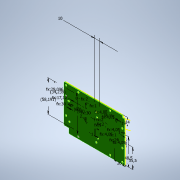
# Autodesk Inventor part: NCU_PCB
Saved by Autodesk Inventor 2021 (Build 250183000, 183)
## iProperties
Created: 2020-02-27
Part Number: NCU_PCB
Material: Generic
Document SubType Name: Modeling
Designer: lgnds
Density: 1 g/cm^3
Appearance: Default
Author: lgnds
Autodesk Inventor part; units mm, degrees
ref_plane "YZ Plane" through (0, 0, 0) normal (1, 0, 0) x (0, 1, 0)
ref_plane "XZ Plane" through (0, 0, 0) normal (0, 1, 0) x (-1, 0, 0)
ref_plane "XY Plane" through (0, 0, 0) normal (0, 0, 1) x (1, 0, 0)
sketch "Sketch1" plane through (0, 0, 0) normal (0, 0, 1) x (1, 0, 0)
  line L0 (-56.1965, -39.8485) -> (56.1965, -39.8485)
  line L1 (56.1965, -39.8485) -> (56.1965, 39.8485)
  line L2 (56.1965, 39.8485) -> (-56.1965, 39.8485)
  line L3 (-56.1965, 39.8485) -> (-56.1965, -39.8485)
  line L4 (-56.1965, -39.8485) -> (56.1965, 39.8485) construction
  line L5 (56.1965, -39.8485) -> (-56.1965, 39.8485) construction
  line L6 (-51.6965, -49.6139) -> (-51.6965, 54.5718) construction
  line L7 (0, -76.4005) -> (0, 76.4005) construction
  line L8 (-3185.9994, 0) -> (3185.9994, 0) construction
  line L9 (-51.6965, 49.6139) -> (-51.6965, -54.5718) construction
  circle A0 centre (-51.6965, -12.8485) radius 1.6
  line L10 (51.6965, -49.6139) -> (51.6965, 54.5718) construction
  line L11 (3185.9994, 0) -> (-3185.9994, 0) construction
  line L12 (51.6965, 49.6139) -> (51.6965, -54.5718) construction
  line L13 (-80.9041, 2.7045) -> (105.3578, 2.7045) construction
  line L14 (51.6965, -49.6139) -> (51.6965, 54.5718) construction
  line L15 (51.6965, 49.6139) -> (51.6965, -54.5718) construction
  circle A1 centre (51.6965, -12.8485) radius 1.6
  circle A2 centre (-51.6965, 18.2575) radius 1.6
  circle A3 centre (51.6965, 18.2575) radius 1.6
  line L16 (-83.6423, -35.3485) -> (68.6664, -35.3485) construction
  circle A4 centre (-29.1965, -35.3485) radius 1.6
  circle A5 centre (29.1965, -35.3485) radius 1.6
  circle A6 centre (-29.1965, 35.3485) radius 1.6
  circle A7 centre (29.1965, 35.3485) radius 1.6
  point P0 (0, 0)
  dimension "d0" = 112.393
  dimension "d1" = 79.697
  dimension "d2" = 4.5
  dimension "d13" = 27
  dimension "d14" = 3.2
  dimension "d15" = 31.106
  dimension "d16" = 4.5
  dimension "d17" = 3.2
  dimension "d18" = 3.2
  dimension "d20" = 27
  dimension "d21" = 27
  constraints: 30 end point, 13 symmetric about line, 8 centre point, 4 point on line, 3 horizontal, 2 midpoint, 2 parallel, 1 perpendicular, 1 vertical, 5 other
  measures "d0" distance of L1.end L2.end
  measures "d1" distance of L0.end L1.end
  measures "d2" distance between parallel lines of L3 L6
  measures "d13" distance from line of L0 A0.centre
  measures "d14" diameter of A0
  measures "d15" distance of A0.centre A2.centre
  measures "d16" distance between parallel lines of L0 L16
  measures "d17" diameter of A4
  measures "d18" diameter of A5
  measures "d20" distance from line of L3 A4.centre
  measures "d21" distance from line of L1 A5.centre
extrude "Extrusion3" add sketch "Sketch1" along normal blind 1.6
thicken "Thicken1" operation add thickness 0.75 both sides no extend neighbours yes toward (0, 1, 0) faces at (-18.7322, -39.8485, 1.0667) (56.1965, -13.2828, 0.5333) (18.7322, 39.8485, 0.5333) (-56.1965, 13.2828, 0.5333)
sketch "Sketch6" plane through (0, 0, 0) normal (0, 0, -1) x (-1, 0, 0)
  circle A0 centre (-5.3535, 12.3015) radius 1.6
  circle A1 centre (46.7956, 12.6015) radius 1.6
  circle A2 centre (45.4465, -19.5985) radius 1.6
  circle A3 centre (-6.7035, -19.8985) radius 1.6
  line L0 (55.4465, 39.0985) -> (55.4465, -39.0985) projected
  line L1 (55.4465, -39.0985) -> (-55.4465, -39.0985) projected
  point P0 (0, 0)
  dimension "d94" = 3.2
  dimension "d95" = 3.2
  dimension "d96" = 3.2
  dimension "d97" = 3.2
  dimension "d98" = 52.15
  dimension "d99" = 52.15
  dimension "d100" = 32.2
  dimension "d102" = 0.3
  dimension "d103" = 32.2
  dimension "d106" = 1.35
  dimension "d107" = 10
  dimension "d108" = 19.5
  constraints: 4 centre point
  measures "d94" diameter of A0
  measures "d95" diameter of A1
  measures "d96" diameter of A3
  measures "d97" diameter of A2
  measures "d98" distance of A0.centre A1.centre
  measures "d99" horizontal distance of A2.centre A3.centre
  measures "d100" vertical distance of A0.centre A3.centre
  measures "d102" vertical distance of A0.centre A1.centre
  measures "d103" vertical distance of A2.centre A1.centre
  measures "d106" horizontal distance of A3.centre A0.centre
  measures "d107" distance from line of L0 A2.centre
  measures "d108" distance from line of L1 A2.centre
extrude "Extrusion6" cut sketch "Sketch6" against normal up to next
sketch "Sketch7" plane through (0, 0, 0) normal (0, 0, -1) x (-1, 0, 0)
  line L0 (-42.5, 39.529) -> (-42.5, 7.5447)
  line L1 (-55.1988, 25) -> (-33.1451, 25)
  line L2 (-55.4465, -39.0985) -> (-55.4465, 39.0985) projected
  line L3 (-55.4465, 39.0985) -> (55.4465, 39.0985) projected
  point P0 (0, 0)
  dimension "d111" = 25
  dimension "d112" = 42.5
  constraints: 4 end point, 1 horizontal, 1 vertical
  measures "d111" distance from line of point (0, 0) L1
  measures "d112" distance from line of point (0, 0) L0
fillet "Fillet3" radius 1 2 edges at (55.4465, -39.0985, 0.8) (-55.4465, 39.0985, 0.8)
sketch "Sketch8" plane through (0, 0, 0) normal (0, 0, -1) x (-1, 0, 0)
  line L0 (55.4465, -39.0985) -> (-54.4465, -39.0985) projected
  line L1 (55.4465, -39.0985) -> (46.4465, -39.0985)
  line L2 (46.4465, -39.0985) -> (46.4465, -30.0985)
  line L3 (46.4465, -30.0985) -> (55.4465, -30.0985)
  line L4 (55.4465, -30.0985) -> (55.4465, -39.0985)
  line L5 (-55.4465, 39.0985) -> (-51.6965, 39.0985)
  line L6 (-51.6965, 39.0985) -> (-51.6965, 35.3485)
  line L7 (-51.6965, 35.3485) -> (-55.4465, 35.3485)
  line L8 (-55.4465, 35.3485) -> (-55.4465, 39.0985)
  point P0 (0, 0)
  dimension "d119" = 9
  dimension "d120" = 9
  dimension "d130" = 3.75
  dimension "d131" = 3.75
  constraints: 16 end point, 4 parallel, 2 horizontal, 2 perpendicular
  measures "d119" distance of L2.end L3.end
  measures "d120" distance of L1.end L2.end
  measures "d130" distance of L5.end L6.end
  measures "d131" distance of L6.end L7.end
extrude "Extrusion7" cut sketch "Sketch8" against normal blind 10
fillet "Fillet5" radius 1 6 edges at (-55.4465, -30.0985, 0.8) (-46.4465, -30.0985, 0.8) (-46.4465, -39.0985, 0.8) (51.6965, 39.0985, 0.8) (51.6965, 35.3485, 0.8) (55.4465, 35.3485, 0.8)
sketch "Sketch9" plane through (0, 0, 0) normal (0, 0, -1) x (-1, 0, 0)
  circle A0 centre (-51.6965, -12.8485) radius 1.6 construction
  circle A1 centre (-29.1965, -35.3485) radius 1.6 construction
  line L0 (-51.6965, -12.8485) -> (-51.6965, -35.3485) construction
  line L1 (-51.6965, -35.3485) -> (-29.1965, -35.3485) construction
  circle A2 centre (29.1965, 35.3485) radius 1.6 construction
  circle A3 centre (51.6965, 18.2575) radius 1.6 construction
  line L2 (29.1965, 35.3485) -> (51.6965, 35.3485) construction
  line L3 (51.6965, 35.3485) -> (51.6965, 18.2575) construction
  circle A4 centre (51.6965, 35.3485) radius 1.6
  circle A5 centre (-51.6965, -35.3485) radius 1.6
  point P0 (0, 0)
  dimension "d124" = 3.2
  dimension "d125" = 3.2
  dimension "d126" = 3.2
  constraints: 8 end point, 2 centre point, 2 coincident, 2 perpendicular, 1 horizontal, 1 vertical
  measures "d124" diameter of A0
  measures "d125" diameter of A5
  measures "d126" diameter of A4
extrude "Extrusion8" cut sketch "Sketch9" against normal up to next
sketch "Sketch10" plane through (0, 0, 0) normal (0, 0, -1) x (-1, 0, 0)
  circle A0 centre (-3.8035, -27.8485) radius 1.6
  line L0 (55.4465, 38.0985) -> (55.4465, -29.0985) projected
  circle A1 centre (-29.1965, 35.3485) radius 1.6 projected
  line L1 (45.4465, -39.0985) -> (-54.4465, -39.0985) projected
  line L2 (-3.8035, -27.8485) -> (-3.8035, 21.0509) construction
  circle A2 centre (-3.8035, 20.1515) radius 1.6
  point P0 (0, 0)
  dimension "d132" = 59.25
  dimension "d133" = 3.2
  dimension "d134" = 3.2
  dimension "d135" = 11.25
  dimension "d136" = 3.2
  dimension "d137" = 48
  constraints: 2 centre point, 2 end point, 1 point on line, 1 vertical
  measures "d132" distance from line of L0 L2.start
  measures "d133" diameter of A0
  measures "d134" diameter of A1
  measures "d135" distance from line of L1 L2.start
  measures "d136" diameter of A2
  measures "d137" distance of A2.centre L2.start
extrude "Extrusion9" cut sketch "Sketch10" against normal up to next contours A0 | A2
sketch "CLIPS" plane through (0, 0, 0) normal (0, 0, -1) x (-1, 0, 0)
  line L0 (-55.4465, -38.0985) -> (-55.4465, 34.3485) projected
  line L1 (-55.4465, 9.4015) -> (-38.9219, 9.4015)
  line L2 (-49.4465, 9.4015) -> (-49.4465, 1.3015)
  line L3 (-36.4465, 30.4761) -> (-36.4465, 19.7209)
  line L4 (-36.4465, 25.0985) -> (-31.2482, 25.0985)
  line L5 (-50.6965, 39.0985) -> (54.4465, 39.0985) projected
  line L6 (1, 31.0993) -> (1, 19.0977)
  line L7 (1, 25.0985) -> (9.1, 25.0985)
  line L8 (-39.6026, -3.5985) -> (-31.2904, -3.5985)
  line L9 (-35.4465, -3.5985) -> (-35.4465, -8.8428)
  line L10 (-12.8208, -3.5985) -> (-5.1792, -3.5985)
  line L11 (-9, -3.5985) -> (-9, -9.7701)
  circle A0 centre (-49.4465, 9.4015) radius 0.5
  circle A1 centre (-35.4465, -3.5985) radius 0.5
  circle A2 centre (-9, -3.5985) radius 0.5
  circle A3 centre (1, 25.0985) radius 0.5
  circle A4 centre (-36.4465, 25.0985) radius 0.5
  circle A5 centre (-49.4465, 5.3515) radius 1
  circle A6 centre (-35.4465, -7.6485) radius 1
  circle A7 centre (-9, -7.6485) radius 1
  circle A8 centre (5.05, 25.0985) radius 1
  circle A9 centre (-32.3965, 25.0985) radius 1
  line L12 (-28.3465, 25.9985) -> (-28.3465, 24.1985) projected
  line L13 (45.4465, -39.0985) -> (-54.4465, -39.0985) projected
  point P0 (0, 0)
  dimension "d140" = 6
  dimension "d141" = 19
  dimension "d142" = 14
  dimension "d143" = 1
  dimension "d144" = 0
  dimension "d145" = 10
  dimension "d146" = 0
  dimension "d147" = 1
  dimension "d148" = 1
  dimension "d149" = 1
  dimension "d150" = 1
  dimension "d151" = 1
  dimension "d157" = 2
  dimension "d158" = 2
  dimension "d159" = 2
  dimension "d160" = 2
  dimension "d161" = 2
  dimension "d162" = 8.1
  dimension "d163" = 4.05
  dimension "d164" = 4.05
  dimension "d165" = 4.05
  dimension "d166" = 4.05
  dimension "d167" = 4.05
  dimension "d168" = 35.5
  dimension "d169" = 48.5
  dimension "d170" = 20
  constraints: 20 end point, 10 centre point, 6 midpoint, 5 coincident, 5 horizontal, 5 point on line, 5 vertical
  measures "d140" distance between parallel lines of L0 L2
  measures "d141" distance between parallel lines of L0 L3
  measures "d142" distance between parallel lines of L5 L4
  measures "d143" distance from line of L6 point (0, 0)
  measures "d144" distance between parallel lines of L4 L7
  measures "d145" distance between parallel lines of L11 L6
  measures "d146" distance between parallel lines of L10 L8
  measures "d147" diameter of A0
  measures "d148" diameter of A1
  measures "d149" diameter of A2
  measures "d150" diameter of A3
  measures "d151" diameter of A4
  measures "d157" diameter of A9
  measures "d158" diameter of A8
  measures "d159" diameter of A7
  measures "d160" diameter of A6
  measures "d161" diameter of A5
  measures "d162" distance between parallel lines of L12 L3
  measures "d163" distance from line of L12 A9.centre
  measures "d164" distance from line of L1 A5.centre
  measures "d165" distance from line of L8 A6.centre
  measures "d166" distance from line of L10 A7.centre
  measures "d167" distance from line of L6 A8.centre
  measures "d168" distance between parallel lines of L13 L8
  measures "d169" distance between parallel lines of L13 L1
  measures "d170" distance between parallel lines of L0 L9
sketch "OUTLINE" plane through (0, 0, 0) normal (0, 0, -1) x (-1, 0, 0)
  line L0 (-50.6965, 39.0985) -> (54.4465, 39.0985) projected
  arc A0 (-50.6965, 39.0985) -> (-51.6965, 38.0985) centre (-50.6965, 38.0985) ccw projected
  line L1 (-51.6965, 38.0985) -> (-51.6965, 36.3485) projected
  arc A1 (-52.6965, 35.3485) -> (-51.6965, 36.3485) centre (-52.6965, 36.3485) ccw projected
  line L2 (-52.6965, 35.3485) -> (-54.4465, 35.3485) projected
  arc A2 (-54.4465, 35.3485) -> (-55.4465, 34.3485) centre (-54.4465, 34.3485) ccw projected
  line L3 (-55.4465, -38.0985) -> (-55.4465, 34.3485) projected
  arc A3 (-55.4465, -38.0985) -> (-54.4465, -39.0985) centre (-54.4465, -38.0985) ccw projected
  line L4 (45.4465, -39.0985) -> (-54.4465, -39.0985) projected
  arc A4 (45.4465, -39.0985) -> (46.4465, -38.0985) centre (45.4465, -38.0985) ccw projected
  line L5 (46.4465, -38.0985) -> (46.4465, -31.0985) projected
  arc A5 (47.4465, -30.0985) -> (46.4465, -31.0985) centre (47.4465, -31.0985) ccw projected
  line L6 (47.4465, -30.0985) -> (54.4465, -30.0985) projected
  arc A6 (54.4465, -30.0985) -> (55.4465, -29.0985) centre (54.4465, -29.0985) ccw projected
  line L7 (55.4465, 38.0985) -> (55.4465, -29.0985) projected
  arc A7 (55.4465, 38.0985) -> (54.4465, 39.0985) centre (54.4465, 38.0985) ccw projected
  point P0 (0, 0)
sketch "EXTRA" plane through (0, 0, 0) normal (0, 0, -1) x (-1, 0, 0)
  circle A0 centre (-29.1965, 35.3485) radius 1.6 projected
  circle A1 centre (-51.6965, 18.2575) radius 1.6 projected
  circle A2 centre (-51.6965, -12.8485) radius 1.6 projected
  circle A3 centre (-51.6965, -35.3485) radius 1.6 projected
  circle A4 centre (-29.1965, -35.3485) radius 1.6 projected
  circle A5 centre (-3.8035, -27.8485) radius 1.5 projected
  circle A6 centre (29.1965, -35.3485) radius 1.5 projected
  circle A7 centre (45.4465, -19.5985) radius 1.6 projected
  circle A8 centre (51.6965, -12.8485) radius 1.5 projected
  circle A9 centre (46.7965, 12.6015) radius 1.6 projected
  circle A10 centre (51.6965, 18.2575) radius 1.5 projected
  circle A11 centre (51.6965, 35.3485) radius 1.6 projected
  circle A12 centre (29.1965, 35.3485) radius 1.6 projected
  circle A13 centre (-5.3535, 12.3015) radius 1.6 projected
  circle A14 centre (-6.7035, -19.8985) radius 1.6 projected
  circle A15 centre (46.7965, 12.6015) radius 1.6 projected
  circle A16 centre (-6.7035, -19.8985) radius 1.6 projected
  circle A17 centre (-5.3535, 12.3015) radius 1.6 projected
  circle A18 centre (45.4465, -19.5985) radius 1.6 projected
  arc A19 (0.0465, -30.6485) -> (3.0465, -33.6485) centre (3.0465, -30.6485) ccw projected
  line L0 (3.0465, -33.6485) -> (37.0465, -33.6485) projected
  arc A20 (37.0465, -33.6485) -> (40.0465, -30.6485) centre (37.0465, -30.6485) ccw projected
  line L1 (40.0465, -30.6485) -> (40.0465, -26.6485) projected
  arc A21 (43.0465, -23.6485) -> (40.0465, -26.6485) centre (43.0465, -26.6485) ccw projected
  line L2 (43.0465, -23.6485) -> (47.0465, -23.6485) projected
  arc A22 (47.0465, -23.6485) -> (50.0465, -20.6485) centre (47.0465, -20.6485) ccw projected
  line L3 (50.0465, -20.6485) -> (50.0465, 13.3515) projected
  arc A23 (50.0465, 13.3515) -> (47.0465, 16.3515) centre (47.0465, 13.3515) ccw projected
  line L4 (47.0465, 16.3515) -> (43.0465, 16.3515) projected
  arc A24 (40.0465, 19.3515) -> (43.0465, 16.3515) centre (43.0465, 19.3515) ccw projected
  line L5 (40.0465, 19.3515) -> (40.0465, 23.3515) projected
  arc A25 (40.0465, 23.3515) -> (37.0465, 26.3515) centre (37.0465, 23.3515) ccw projected
  line L6 (37.0465, 26.3515) -> (3.0465, 26.3515) projected
  arc A26 (3.0465, 26.3515) -> (0.0465, 23.3515) centre (3.0465, 23.3515) ccw projected
  line L7 (0.0465, 23.3515) -> (0.0465, 19.3515) projected
  arc A27 (-2.9535, 16.3515) -> (0.0465, 19.3515) centre (-2.9535, 19.3515) ccw projected
  line L8 (-2.9535, 16.3515) -> (-6.9535, 16.3515) projected
  arc A28 (-6.9535, 16.3515) -> (-9.9535, 13.3515) centre (-6.9535, 13.3515) ccw projected
  line L9 (-9.9535, 13.3515) -> (-9.9535, -20.6485) projected
  arc A29 (-9.9535, -20.6485) -> (-6.9535, -23.6485) centre (-6.9535, -20.6485) ccw projected
  line L10 (-6.9535, -23.6485) -> (-2.9535, -23.6485) projected
  arc A30 (0.0465, -26.6485) -> (-2.9535, -23.6485) centre (-2.9535, -26.6485) ccw projected
  line L11 (0.0465, -26.6485) -> (0.0465, -30.6485) projected
  line L12 (-40.0752, 37.0701) -> (-38.5847, 33.693) projected
  line L13 (-40.0752, 37.0701) -> (-38.5847, 33.693) projected
  arc A31 (-40.0752, 37.0701) -> (-44.924, 37.0701) centre (-42.4996, 36.0001) ccw projected
  line L14 (-46.4144, 33.693) -> (-44.924, 37.0701) projected
  arc A32 (-46.4144, 33.693) -> (-46.4996, 33.2892) centre (-45.4996, 33.2892) ccw projected
  line L15 (-46.4996, 33.2892) -> (-46.4996, 32.3001) projected
  arc A33 (-38.4996, 33.2892) -> (-38.5847, 33.693) centre (-39.4996, 33.2892) ccw projected
  line L16 (-38.4996, 32.3001) -> (-38.4996, 33.2892) projected
  line L17 (-38.5847, 16.3072) -> (-40.0752, 12.9301) projected
  line L18 (-38.5847, 16.3072) -> (-40.0752, 12.9301) projected
  arc A34 (-38.5847, 16.3072) -> (-38.4996, 16.7109) centre (-39.4996, 16.7109) ccw projected
  line L19 (-38.4996, 16.7109) -> (-38.4996, 17.7001) projected
  arc A35 (-44.924, 12.9301) -> (-40.0752, 12.9301) centre (-42.4996, 14.0001) ccw projected
  line L20 (-44.924, 12.9301) -> (-46.4144, 16.3072) projected
  arc A36 (-46.4996, 16.7109) -> (-46.4144, 16.3072) centre (-45.4996, 16.7109) ccw projected
  line L21 (-46.4996, 17.7001) -> (-46.4996, 16.7109) projected
  line L22 (-47, 25.875) -> (-47, 24.125) projected
  line L23 (-38.4996, 23.7001) -> (-38.4996, 26.3001) projected
  arc A37 (-38, 32.8725) -> (-38.3482, 33.3489) centre (-38.5, 32.8725) ccw projected
  arc A38 (-38.3482, 16.6511) -> (-38, 17.1275) centre (-38.5, 17.1275) ccw projected
  line L24 (-37.9731, 17.7501) -> (-37.9731, 32.2501) projected
  circle A39 centre (-43.9996, 31.0001) radius 0.49 projected
  circle A40 centre (-40.9996, 19.0001) radius 0.49 projected
  line L25 (18.1639, 29.2483) -> (38.1791, 29.2483) projected
  line L26 (18.1639, 29.2483) -> (38.1791, 29.2483) projected
  line L27 (18.1639, 29.2483) -> (38.1791, 29.2483) projected
  arc A41 (18.1639, 29.2483) -> (11.0519, 22.1363) centre (18.1639, 22.1363) ccw projected
  line L28 (11.0519, -21.8311) -> (11.0519, 22.1363) projected
  arc A42 (11.0519, -21.8311) -> (18.1639, -28.9431) centre (18.1639, -21.8311) ccw projected
  line L29 (38.1791, -28.9431) -> (18.1639, -28.9431) projected
  arc A43 (38.1791, -28.9431) -> (45.2911, -21.8311) centre (38.1791, -21.8311) ccw projected
  line L30 (45.2911, 22.1363) -> (45.2911, -21.8311) projected
  arc A44 (45.2911, 22.1363) -> (38.1791, 29.2483) centre (38.1791, 22.1363) ccw projected
  line L31 (-47.9731, 16.7501) -> (-38.9731, 16.7501) projected
  line L32 (-64.4731, 20.5981) -> (-47.9731, 16.7501) projected
  line L33 (-47.9731, 33.2501) -> (-64.4731, 37.0981) projected
  line L34 (-38.9731, 33.2501) -> (-47.9731, 33.2501) projected
  arc A45 (-37.9731, 32.2501) -> (-38.9731, 33.2501) centre (-38.9731, 32.2501) ccw projected
  arc A46 (-38.9731, 16.7501) -> (-37.9731, 17.7501) centre (-38.9731, 17.7501) ccw projected
  circle A47 centre (23.6122, 11.2651) radius 0.7836 projected
  circle A48 centre (32.7308, -10.9599) radius 0.7836 projected
  circle A49 centre (20.0465, -3.6485) radius 1
  circle A50 centre (28.1715, 0.1526) radius 1
  circle A51 centre (-3.8035, 20.1515) radius 1.6 projected
  point P0 (0, 0)
  dimension "d152" = 2
  dimension "d153" = 30
  dimension "d154" = 60
  dimension "d155" = 60
  dimension "d156" = 30
  dimension "d171" = 2
  dimension "d173" = 58.1914
  dimension "d174" = 34.2392
  dimension "d175" = 17.1196
  dimension "d176" = 29.0957
  constraints: 2 centre point
  measures "d152" diameter of A49
  measures "d153" distance from line of L6 A49.centre
  measures "d154" distance between parallel lines of L6 L0
  measures "d155" distance between parallel lines of L3 L9
  measures "d156" distance from line of L3 A49.centre
  measures "d171" diameter of A50
  measures "d173" distance between parallel lines of L29 L25
  measures "d174" distance between parallel lines of L30 L28
  measures "d175" distance from line of L30 A50.centre
  measures "d176" distance from line of L25 A50.centre
equation "\"d16\" = d2"
equation "\"d17\" = d14"
equation "\"d18\" = d14"
equation "\"d20\" = d13"
equation "\"d21\" = d20"
equation "\"d95\" = d94"
equation "\"d96\" = d94"
equation "\"d97\" = d94"
equation "\"d103\" = d100"
equation "\"d120\" = d119"
equation "\"d131\" = d130"
equation "\"d125\" = d124"
equation "\"d126\" = d124"
equation "\"d133\" = d134"
equation "\"d136\" = d134"
body "Solid2"
